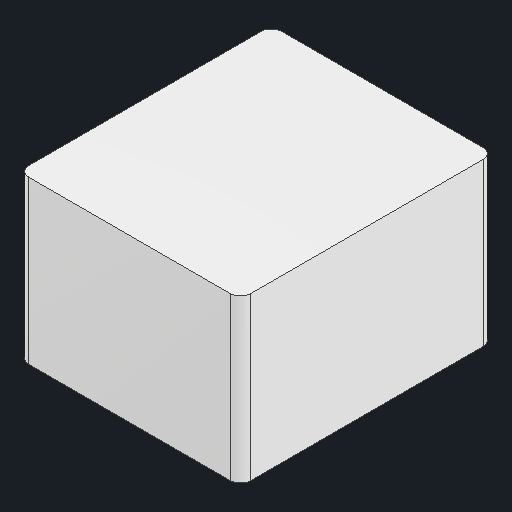
# Autodesk Inventor part: encloser_valve-solenoid
Saved by Autodesk Inventor 2025.2 (Build 292293000, 293)
## iProperties
Created: 2026-01-02
Part Number: encloser_valve-solenoid
Material: ABS Plastic
Document SubType Name: Modeling
Designer: sam
Density: 1.06 g/cm^3
Appearance: Smooth - White
Author: sam
Autodesk Inventor part; units mm, degrees
ref_plane "YZ Plane" through (0, 0, 0) normal (1, 0, 0) x (0, 1, 0)
ref_plane "XZ Plane" through (0, 0, 0) normal (0, 1, 0) x (-1, 0, 0)
ref_plane "XY Plane" through (0, 0, 0) normal (0, 0, 1) x (1, 0, 0)
sketch "Sketch1" plane through (0, 0, 0) normal (0, 1, 0) x (-1, 0, 0)
  line L0 (21.5, 24.5) -> (-21.5, 24.5)
  line L1 (-21.5, 24.5) -> (-21.5, -24.5)
  line L2 (-21.5, -24.5) -> (21.5, -24.5)
  line L3 (21.5, -24.5) -> (21.5, 24.5)
  line L4 (21.5, 24.5) -> (-21.5, -24.5) construction
  line L5 (-21.5, 24.5) -> (21.5, -24.5) construction
  point P0 (0, 0)
  dimension "d0" = 43
  dimension "d1" = 49
  constraints: 12 end point, 2 midpoint, 2 parallel, 1 horizontal, 1 perpendicular
  measures "d0" distance of L2.end L1.end
  measures "d1" distance of L1.end L0.end
extrude "Extrusion1" add sketch "Sketch1" against normal blind 2
sketch "Sketch2" plane through (0, -2, 0) normal (0, -1, 0) x (1, 0, 0)
  line L0 (21.5, -24.5) -> (21.5, 24.5) projected
  line L1 (21.5, 24.5) -> (-21.5, 24.5) projected
  line L2 (-21.5, 24.5) -> (-21.5, -24.5) projected
  line L3 (-21.5, -24.5) -> (21.5, -24.5) projected
  line L4 (-21.5, 24.5) -> (-18.2, 24.5)
  line L5 (-18.2, 24.5) -> (-18.2, -24.5)
  line L6 (-18.2, -24.5) -> (-21.5, -24.5)
  line L7 (-21.5, -24.5) -> (-21.5, 24.5)
  line L8 (21.5, 24.5) -> (18.2, 24.5)
  line L9 (18.2, 24.5) -> (18.2, -24.5)
  line L10 (18.2, -24.5) -> (21.5, -24.5)
  line L11 (21.5, -24.5) -> (21.5, 24.5)
  line L12 (-18.2, 24.5) -> (18.2, 24.5)
  line L13 (18.2, 24.5) -> (18.2, 16)
  line L14 (18.2, 16) -> (-18.2, 16)
  line L15 (-18.2, 16) -> (-18.2, 24.5)
  line L16 (18.2, -24.5) -> (-18.2, -24.5)
  line L17 (-18.2, -24.5) -> (-18.2, -20.9)
  line L18 (-18.2, -20.9) -> (18.2, -20.9)
  line L19 (18.2, -20.9) -> (18.2, -24.5)
  point P0 (0, 0)
  point P1 (-18.2, 16)
  point P2 (18.2, -20.9)
  dimension "d4" = 3.3
  dimension "d5" = 3.3
  dimension "d6" = 8.5
  dimension "d7" = 3.6
  constraints: 32 end point, 8 parallel, 4 horizontal, 4 perpendicular, 4 point on line
  measures "d4" distance of L5.end L6.end
  measures "d5" distance of L10.end L9.end
  measures "d6" distance of L12.end L13.end
  measures "d7" distance of L16.end L17.end
extrude "Extrusion2" add sketch "Sketch2" along normal blind 29.4 contours L3 L9 L1 L0 | L3 L5 L18 L9 | L9 L14 L5 L1 | L3 L2 L1 L5
sketch "Sketch3" plane through (-21.5, 0, 24.5) normal (0, 0, 1) x (1, 0, 0)
  line L0 (0, 0) -> (43, 0) projected
  line L1 (0, 0) -> (0, -31.4) projected
  line L2 (43, -31.4) -> (0, -31.4) projected
  line L3 (43, 0) -> (43, -31.4) projected
  line L4 (10.7, -31.4) -> (32.3, -31.4)
  line L5 (32.3, -31.4) -> (32.3, -5.6)
  line L6 (32.3, -5.6) -> (10.7, -5.6)
  line L7 (10.7, -5.6) -> (10.7, -31.4)
  point P0 (21.5, 0)
  point P1 (21.5, -31.4)
  dimension "d12" = 21.6
  dimension "d13" = 25.8
  dimension "d14" = 10.8
  constraints: 8 end point, 2 parallel, 1 horizontal, 1 midpoint, 1 perpendicular, 1 point on line
  measures "d12" distance of L6.end L5.end
  measures "d13" distance between parallel lines of L2 L6
  measures "d14" distance from line of point (21.5, -31.4) L7
extrude "Extrusion3" cut sketch "Sketch3" along normal blind 10 from surface at -49 contours L7 L6 L5 L2
fillet "Fillet1" radius 2 4 edges at (21.5, -15.7, 24.5) (21.5, -15.7, -24.5) (-21.5, -15.7, 24.5) (-21.5, -15.7, -24.5)
equation "\"d14\" = 0.5 * d12"
body "Solid1"
